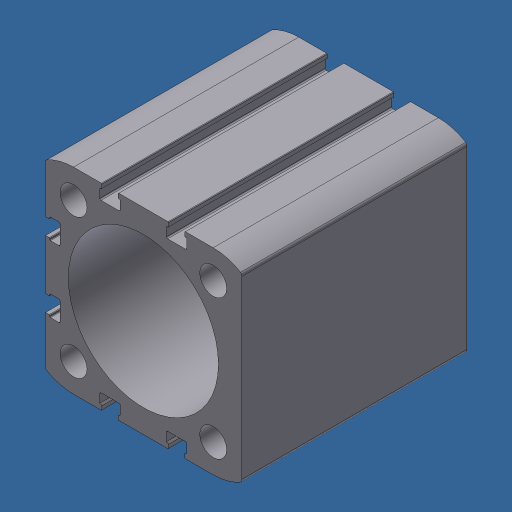
# Autodesk Inventor part: EXTRUSION,CYLINDER, ALUMINIUM, FESTO, 50MM
Saved by Autodesk Inventor 2024.3 (Build 283343000, 343)
## iProperties
Manager: _
Category: _
RuleStatus: InUse
Shininess: 64.0
Angle Display Precision: 2
Document Length Units: 11269
Document Angle Units: 11279
Document Time Units: 11290
Document Mass Units: 11283
Document Length Units Precision: 3
Document Angle Units Precision: 2
Part Number: EXTRUSION,CYLINDER, ALUMINIUM, FESTO, 50MM
Material: Aluminum, 6061-T6
Document SubType Name: Modeling
Created: 2019-07-31
Designer: -
Manufacturer: Standard
Standards Organization: Custom
Checked By: 00
Engr Approved By: _
User Status: Work In Process
Description: EXTRUSION, CYLINDER, ALUMINIUM, FESTO, 50MM
Density: 2.71 g/cm^3
Mfg Approved By: -
Appearance: Aluminum (Flat)
BeforeDocSave0: Mass
BeforeDocSave1: PartFinishTrigger
Density: 0.0
Volumn: 0.0
Area: 0.0
PropertySet Name: Model Information
Control State: 0
Master: False
Checked Out: False
CN_MASS: 0.38
CN_SERVICEABLE: _
CL_runCount: 0
FIRST_DESCRIPTION: _
SECOND_DESCRIPTION: _
THIRD_DESCRIPTION: _
Revision Number: A
Subject: _
Author: -
Keywords: -
Autodesk Inventor part; units mm, degrees
ref_plane "YZ Plane" through (0, 0, 0) normal (1, 0, 0) x (0, 1, 0)
ref_plane "XZ Plane" through (0, 0, 0) normal (0, 1, 0) x (-1, 0, 0)
ref_plane "XY Plane" through (0, 0, 0) normal (0, 0, 1) x (1, 0, 0)
sketch "Sketch1" plane through (0, 0, 0) normal (0, 0, 1) x (1, 0, 0)
  line L0 (0, 53.3773) -> (0, -40.0186) projected
  line L1 (-39.496, 0) -> (52.7454, 0) projected
  line L2 (-23.25, 32.75) -> (-14.7105, 32.75)
  line L3 (-13.8, 32.55) -> (-13.8, 31.35)
  line L4 (-14.5, 30.95) -> (-14.5, 28.15)
  line L5 (-14.1, 27.75) -> (-8.1, 27.75)
  line L6 (-7.7, 28.15) -> (-7.7, 30.95)
  line L7 (-8.4, 31.35) -> (-8.4, 32.55)
  line L8 (8.4, 32.55) -> (8.4, 31.35)
  line L9 (8.1659, 31.15) -> (7.9, 31.15)
  line L10 (7.7, 30.95) -> (7.7, 28.15)
  line L11 (8.1, 27.75) -> (14.1, 27.75)
  line L12 (14.5, 28.15) -> (14.5, 30.95)
  line L13 (13.8, 31.35) -> (13.8, 32.55)
  line L14 (32.75, 29.2025) -> (32.75, -29.3325)
  line L15 (23.25, -32.75) -> (14.3148, -32.75)
  line L16 (13.8, -32.55) -> (13.8, -31.35)
  line L17 (14.0222, -31.15) -> (14.3, -31.15)
  line L18 (14.5, -30.95) -> (14.5, -28.15)
  line L19 (14.1, -27.75) -> (8.1, -27.75)
  line L20 (7.7, -28.15) -> (7.7, -30.95)
  line L21 (8.4, -31.35) -> (8.4, -32.55)
  line L22 (-8.4, -32.55) -> (-8.4, -31.35)
  line L23 (-8.2, -31.15) -> (-7.9, -31.15)
  line L24 (-7.7, -30.95) -> (-7.7, -28.15)
  line L25 (-8.1, -27.75) -> (-14.1, -27.75)
  line L26 (-14.5, -28.15) -> (-14.5, -30.95)
  line L27 (-13.8, -31.35) -> (-13.8, -32.55)
  line L28 (-32.75, -29.3354) -> (-32.75, -14)
  line L29 (-32.55, -13.8) -> (-31.35, -13.8)
  line L30 (-30.95, -14.5) -> (-28.15, -14.5)
  line L31 (-27.75, -14.1) -> (-27.75, -8.1)
  line L32 (-28.15, -7.7) -> (-30.95, -7.7)
  line L33 (-31.35, -8.4) -> (-32.55, -8.4)
  line L34 (-32.55, 8.4) -> (-31.35, 8.4)
  line L35 (-31.15, 8.2) -> (-31.15, 7.9)
  line L36 (-30.95, 7.7) -> (-28.15, 7.7)
  line L37 (-27.75, 8.1) -> (-27.75, 14.1)
  line L38 (-28.15, 14.5) -> (-30.95, 14.5)
  line L39 (-31.15, 14.3) -> (-31.15, 14)
  line L40 (-31.35, 13.8) -> (-32.55, 13.8)
  arc A0 (-23.25, 32.75) -> (-32.201, 30.3542) centre (-23.255, 14.85) ccw
  arc A1 (32.3753, 30.2493) -> (23.25, 32.75) centre (23.25, 14.85) ccw
  arc A2 (32.1403, -30.3862) -> (32.75, -29.3325) centre (31.65, -29.3992) ccw
  arc A3 (32.75, 29.2025) -> (32.0235, 30.4524) centre (31.65, 29.3992) ccw
  arc A4 (-32.201, 30.3542) -> (-32.75, 29.3248) centre (-31.65, 29.3992) ccw
  arc A5 (-32.75, -29.3354) -> (-32.1428, -30.3847) centre (-31.65, -29.3992) ccw
  arc A6 (-32.257, -30.3188) -> (-23.25, -32.75) centre (-23.25, -14.85) ccw
  arc A7 (23.25, -32.75) -> (32.2596, -30.3173) centre (23.25, -14.85) ccw
  line L41 (-32.75, 14) -> (-32.75, 29.3248)
  line L42 (-31.15, -7.9) -> (-31.15, -8.2)
  line L43 (-31.15, -14) -> (-31.15, -14.3)
  line L44 (-32.75, -8.2) -> (-32.75, 8.2)
  line L45 (-14.3, -31.15) -> (-14, -31.15)
  line L46 (-14, -32.75) -> (-23.25, -32.75)
  line L47 (14.3148, -32.75) -> (14, -32.75)
  line L48 (8.2, -32.75) -> (-8.2, -32.75)
  line L49 (7.9, -31.15) -> (8.2, -31.15)
  line L50 (14, -31.15) -> (14.0222, -31.15)
  line L51 (7.8505, 32.75) -> (8.2, 32.75)
  line L52 (14, 32.75) -> (23.25, 32.75)
  line L53 (14.3, 31.15) -> (14, 31.15)
  line L54 (8.2, 31.15) -> (8.1659, 31.15)
  line L55 (-14.7105, 32.75) -> (-14, 32.75)
  line L56 (-8.2, 32.75) -> (7.8505, 32.75)
  line L57 (-7.9, 31.15) -> (-8.2, 31.15)
  line L58 (-14, 31.15) -> (-14.0144, 31.15)
  circle A8 centre (0, 0) radius 25
  arc A9 (-13.8, 32.55) -> (-14, 32.75) centre (-14, 32.55) ccw
  arc A10 (-14, 31.15) -> (-13.8, 31.35) centre (-14, 31.35) ccw
  arc A11 (-14.3, 31.15) -> (-14.5, 30.95) centre (-14.3, 30.95) ccw
  arc A12 (-8.4, 31.35) -> (-8.2, 31.15) centre (-8.2, 31.35) ccw
  arc A13 (-7.7, 30.95) -> (-7.9, 31.15) centre (-7.9, 30.95) ccw
  arc A14 (-8.2, 32.75) -> (-8.4, 32.55) centre (-8.2, 32.55) ccw
  line L59 (-14.3, 31.15) -> (-14, 31.15)
  arc A15 (8.4, 32.55) -> (8.2, 32.75) centre (8.2, 32.55) ccw
  arc A16 (8.2, 31.15) -> (8.4, 31.35) centre (8.2, 31.35) ccw
  arc A17 (7.9, 31.15) -> (7.7, 30.95) centre (7.9, 30.95) ccw
  arc A18 (14.5, 30.95) -> (14.3, 31.15) centre (14.3, 30.95) ccw
  arc A19 (13.8, 31.35) -> (14, 31.15) centre (14, 31.35) ccw
  arc A20 (14, 32.75) -> (13.8, 32.55) centre (14, 32.55) ccw
  arc A21 (-32.75, 14) -> (-32.55, 13.8) centre (-32.55, 14) ccw
  arc A22 (-31.35, 13.8) -> (-31.15, 14) centre (-31.35, 14) ccw
  arc A23 (-30.95, 14.5) -> (-31.15, 14.3) centre (-30.95, 14.3) ccw
  arc A24 (-31.15, 7.9) -> (-30.95, 7.7) centre (-30.95, 7.9) ccw
  arc A25 (-31.15, 8.2) -> (-31.35, 8.4) centre (-31.35, 8.2) ccw
  arc A26 (-32.55, 8.4) -> (-32.75, 8.2) centre (-32.55, 8.2) ccw
  arc A27 (-30.95, -7.7) -> (-31.15, -7.9) centre (-30.95, -7.9) ccw
  arc A28 (-31.35, -8.4) -> (-31.15, -8.2) centre (-31.35, -8.2) ccw
  arc A29 (-32.75, -8.2) -> (-32.55, -8.4) centre (-32.55, -8.2) ccw
  arc A30 (-31.15, -14.3) -> (-30.95, -14.5) centre (-30.95, -14.3) ccw
  arc A31 (-31.15, -14) -> (-31.35, -13.8) centre (-31.35, -14) ccw
  arc A32 (-32.55, -13.8) -> (-32.75, -14) centre (-32.55, -14) ccw
  arc A33 (-14, -32.75) -> (-13.8, -32.55) centre (-14, -32.55) ccw
  arc A34 (-13.8, -31.35) -> (-14, -31.15) centre (-14, -31.35) ccw
  arc A35 (-14.5, -30.95) -> (-14.3, -31.15) centre (-14.3, -30.95) ccw
  arc A36 (-8.2, -31.15) -> (-8.4, -31.35) centre (-8.2, -31.35) ccw
  arc A37 (-7.9, -31.15) -> (-7.7, -30.95) centre (-7.9, -30.95) ccw
  arc A38 (-8.4, -32.55) -> (-8.2, -32.75) centre (-8.2, -32.55) ccw
  arc A39 (8.2, -32.75) -> (8.4, -32.55) centre (8.2, -32.55) ccw
  arc A40 (8.4, -31.35) -> (8.2, -31.15) centre (8.2, -31.35) ccw
  arc A41 (7.7, -30.95) -> (7.9, -31.15) centre (7.9, -30.95) ccw
  arc A42 (14.3, -31.15) -> (14.5, -30.95) centre (14.3, -30.95) ccw
  arc A43 (14, -31.15) -> (13.8, -31.35) centre (14, -31.35) ccw
  arc A44 (13.8, -32.55) -> (14, -32.75) centre (14, -32.55) ccw
  arc A45 (14.5, -28.15) -> (14.1, -27.75) centre (14.1, -28.15) ccw
  arc A46 (8.1, -27.75) -> (7.7, -28.15) centre (8.1, -28.15) ccw
  arc A47 (-7.7, -28.15) -> (-8.1, -27.75) centre (-8.1, -28.15) ccw
  arc A48 (-14.1, -27.75) -> (-14.5, -28.15) centre (-14.1, -28.15) ccw
  arc A49 (-28.15, -14.5) -> (-27.75, -14.1) centre (-28.15, -14.1) ccw
  arc A50 (-27.75, -8.1) -> (-28.15, -7.7) centre (-28.15, -8.1) ccw
  arc A51 (-28.15, 7.7) -> (-27.75, 8.1) centre (-28.15, 8.1) ccw
  arc A52 (-27.75, 14.1) -> (-28.15, 14.5) centre (-28.15, 14.1) ccw
  arc A53 (-14.5, 28.15) -> (-14.1, 27.75) centre (-14.1, 28.15) ccw
  arc A54 (-8.1, 27.75) -> (-7.7, 28.15) centre (-8.1, 28.15) ccw
  arc A55 (7.7, 28.15) -> (8.1, 27.75) centre (8.1, 28.15) ccw
  arc A56 (14.1, 27.75) -> (14.5, 28.15) centre (14.1, 28.15) ccw
  point P0 (-13.8, 32.75)
  point P1 (-13.8, 31.15)
  point P2 (-14.5, 27.75)
  point P3 (-7.7, 27.75)
  point P4 (-7.7, 31.15)
  point P5 (-8.4, 31.15)
  point P6 (-8.4, 32.75)
  point P7 (8.4, 32.75)
  point P8 (8.4, 31.15)
  point P9 (7.7, 31.15)
  point P10 (7.7, 27.75)
  point P11 (14.5, 27.75)
  point P12 (14.5, 31.15)
  point P13 (13.8, 31.15)
  point P14 (13.8, 32.75)
  point P15 (13.8, -32.75)
  point P16 (13.8, -31.15)
  point P17 (14.5, -31.15)
  point P18 (14.5, -27.75)
  point P19 (7.7, -27.75)
  point P20 (7.7, -31.15)
  point P21 (8.4, -31.15)
  point P22 (8.4, -32.75)
  point P23 (-8.4, -32.75)
  point P24 (-8.4, -31.15)
  point P25 (-7.7, -27.75)
  point P26 (-14.5, -27.75)
  point P27 (-14.5, -31.15)
  point P28 (-13.8, -31.15)
  point P29 (-13.8, -32.75)
  point P30 (-32.75, -13.8)
  point P31 (-31.15, -13.8)
  point P32 (-31.15, -14.5)
  point P33 (-27.75, -14.5)
  point P34 (-27.75, -7.7)
  point P35 (-31.15, -7.7)
  point P36 (-31.15, -8.4)
  point P37 (-32.75, -8.4)
  point P38 (-32.75, 8.4)
  point P39 (-31.15, 8.4)
  point P40 (-31.15, 7.7)
  point P41 (-27.75, 7.7)
  point P42 (-27.75, 14.5)
  point P43 (-31.15, 14.5)
  point P44 (-31.15, 13.8)
  point P45 (-32.75, 13.8)
  point P46 (-7.7, -31.15)
  dimension "d0" = 35.8
  dimension "d1" = 50
  dimension "d4" = 0.2
  dimension "d5" = 0.2
  dimension "d6" = 0.4
  constraints: 120 point on circle, 116 end point, 98 tangent, 94 point on line, 57 centre point, 46 equal radius, 31 horizontal, 26 vertical, 1 coincident, 1 collinear, 8 other
  measures "d0" diameter of A0
  measures "d1" diameter of A8
  measures "d4" radius of A9
  measures "d5" radius of A15
  measures "d6" radius of A45
extrude "FESTO, 50MM" add sketch "Sketch1" against normal blind 75 contours L56 L51 A15 L8 A16 L54 L9 A17 L10 A55 L11 A56 L12 A18 L53 A19 L13 A20 L52 A1 A3 L14 L1 A8 L0 | L0 A8 L1 L44 A26 L34 A25 L35 A24 L36 A51 L37 A52 L38 A23 L39 A22 L40 A21 L41 A4 A0 L2 L55 A9 L3 A10 L58 L59 A11 L4 A53 L5 A54 L6 A13 L57 A12 L7 A14 L56 | L1 L14 A2 A7 L15 L47 A44 L16 A43 L50 L17 A42 L18 A45 L19 A46 L20 A41 L49 A40 L21 A39 L48 L0 A8 | A8 L0 L48 A38 L22 A36 L23 A37 L24 A47 L25 A48 L26 A35 L45 A34 L27 A33 L46 A6 A5 L28 A32 L29 A31 L43 A30 L30 A49 L31 A50 L32 A27 L42 A28 L33 A29 L44 L1
sketch "Sketch2" plane through (0, 0, 0) normal (0, 0, 1) x (1, 0, 0)
  line L0 (0, 52.4) -> (0, -39.3) projected
  line L1 (-39.3045, 0) -> (52.4235, 0) projected
  point P0 (-23.25, 23.25)
  point P1 (23.25, 23.25)
  point P2 (23.25, -23.25)
  point P3 (-23.25, -23.25)
  dimension "d7" = 23.25
  dimension "d8" = 23.25
  dimension "d9" = 23.25
  dimension "d10" = 23.25
  constraints: 2 horizontal alignment, 2 vertical alignment
  measures "d7" distance from line of point (-23.25, 23.25) L0
  measures "d8" distance from line of point (23.25, 23.25) L0
  measures "d9" distance from line of point (-23.25, 23.25) L1
  measures "d10" distance from line of L1 point (-23.25, -23.25)
hole "Hole1" at (-23.25, 23.25, 0) at (23.25, 23.25, 0) at (23.25, -23.25, 0) at (-23.25, -23.25, 0) direction (0, 0, -1) diameter 9 end through all
equation "\"d8\" = d7"
equation "\"d9\" = d7"
equation "\"d10\" = d7"
